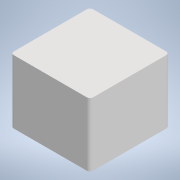
# Autodesk Inventor part: stepper driver
Saved by Autodesk Inventor 2020 (Build 240168000, 168)
## iProperties
Created: 2022-12-14
Part Number: stepper driver
Material: Generic
Document SubType Name: Modeling
Designer: Manish
Density: 1 g/cm^3
Appearance: Default
Author: Manish
Autodesk Inventor part; units mm, degrees
ref_plane "YZ Plane" through (0, 0, 0) normal (1, 0, 0) x (0, 1, 0)
ref_plane "XZ Plane" through (0, 0, 0) normal (0, 1, 0) x (-1, 0, 0)
ref_plane "XY Plane" through (0, 0, 0) normal (0, 0, 1) x (1, 0, 0)
sketch "Sketch1" plane through (0, 0, 0) normal (0, 1, 0) x (-1, 0, 0)
  line L0 (-2, 0) -> (-48, 0)
  line L1 (-50, -2) -> (-50, -48)
  line L2 (-48, -50) -> (-2, -50)
  line L3 (0, -48) -> (0, -2)
  arc A0 (0, -2) -> (-2, 0) centre (-2, -2) ccw
  arc A1 (-50, -48) -> (-48, -50) centre (-48, -48) ccw
  arc A2 (-2, -50) -> (0, -48) centre (-2, -48) ccw
  arc A3 (-48, 0) -> (-50, -2) centre (-48, -2) ccw
  point P0 (0, 0)
  point P1 (-50, 0)
  point P2 (-50, -50)
  dimension "d0" = 50
  dimension "d1" = 50
  dimension "d2" = 2
  constraints: 8 end point, 8 point on circle, 8 tangent, 6 point on line, 4 centre point, 3 equal radius, 2 parallel, 1 horizontal, 1 perpendicular
  measures "d0" distance of point (0, 0) point (-50, 0)
  measures "d1" distance of point (-50, -50) point (-50, 0)
  measures "d2" radius of A0
extrude "Extrusion1" add sketch "Sketch1" along normal blind 40
body "Solid1"
